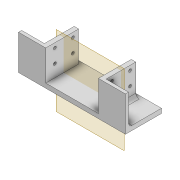
# Autodesk Inventor part: Motor_test_mount
Saved by Autodesk Inventor 2022 (Build 260153000, 153)
## iProperties
Created: 2022-05-04
Part Number: Motor_test_mount
Material: Generic
Document SubType Name: Modeling
Designer: dell
Density: 1 g/cm^3
Appearance: Default
Author: dell
Autodesk Inventor part; units mm, degrees
ref_plane "YZ Plane" through (0, 0, 0) normal (1, 0, 0) x (0, 1, 0)
ref_plane "XZ Plane" through (0, 0, 0) normal (0, 1, 0) x (-1, 0, 0)
ref_plane "XY Plane" through (0, 0, 0) normal (0, 0, 1) x (1, 0, 0)
sketch "Sketch2" plane through (0, 0, 0) normal (1, 0, 0) x (0, 1, 0)
  line L0 (26.4, -3) -> (6, -3)
  line L1 (6, -3) -> (6, -23.4)
  line L2 (6, -23.4) -> (26.4, -23.4)
  line L3 (26.4, -23.4) -> (26.4, -3)
  line L4 (30.4, 0) -> (0, 0)
  line L5 (30.4, -26.4) -> (30.4, 0)
  line L6 (0, 0) -> (0, -26.4)
  line L7 (30.4, -26.4) -> (0, -26.4)
  line L8 (6, -11) -> (0, -11)
  line L9 (0, -11) -> (0, -15.4)
  line L10 (0, -15.4) -> (6, -15.4)
  line L11 (6, -15.4) -> (6, -11)
  point P0 (0, -11)
  dimension "d5" = 20.4
  dimension "d6" = 20.4
  dimension "d8" = 6
  dimension "d22" = 4
  dimension "d23" = 3
  dimension "d24" = 3
  dimension "d27" = 8
  dimension "d28" = 8
  constraints: 24 end point, 4 parallel, 3 horizontal, 2 perpendicular, 2 point on line, 1 coincident, 1 vertical
  measures "d5" distance of L0.start L0.end
  measures "d6" distance of L0.end L1.end
  measures "d8" distance between parallel lines of L1 L6
  measures "d22" distance between parallel lines of L5 L3
  measures "d23" distance between parallel lines of L2 L7
  measures "d24" distance between parallel lines of L4 L0
  measures "d27" distance from line of L0.end L8
  measures "d28" distance from line of L1.end L10
extrude "Extrusion1" add sketch "Sketch2" along normal blind 54.8 contours L0 L1 L8 L6 L4 L5 L7 L10 L2 L3
sketch "Sketch13" plane through (0, 30.4, 0) normal (0, 1, 0) x (1, 0, 0)
  line L0 (0, 0) -> (54.8, 0) projected
  line L1 (0, 26.4) -> (54.8, 26.4) projected
  line L2 (54.8, 0) -> (50.8, 0)
  line L3 (50.8, 0) -> (50.8, 26.4)
  line L4 (50.8, 26.4) -> (54.8, 26.4)
  line L5 (54.8, 26.4) -> (54.8, 0)
  line L6 (4, 0) -> (0, 0)
  line L7 (0, 0) -> (0, 26.4)
  line L8 (0, 26.4) -> (4, 26.4)
  line L9 (4, 26.4) -> (4, 0)
  line L10 (0, 26.4) -> (0, 0) projected
  point P0 (0, 0)
  point P1 (69.8, 0)
  point P2 (69.8, 26.4)
  point P3 (4, 0)
  point P4 (54.8, 26.4)
  point P5 (50.8, 0)
  dimension "d75" = 4
  dimension "d76" = 4
  dimension "d77" = 46.8
  constraints: 17 end point, 4 parallel, 3 point on line, 2 horizontal, 2 perpendicular, 1 collinear
  measures "d75" distance between parallel lines of L5 L3
  measures "d76" distance between parallel lines of L9 L7
  measures "d77" distance between parallel lines of L3 L9
extrude "Extrusion11" add sketch "Sketch13" along normal blind 27 contours L7 L1 L9 L0 | L3 L1 L5 L0
sketch "Sketch14" plane through (54.8, 30.4, 0) normal (1, 0, 0) x (0, 0, -1)
  circle A0 centre (5.2, 11) radius 1.3
  circle A1 centre (5.2, 23) radius 1.3
  line L0 (0, -30.4) -> (0, 27) projected
  circle A2 centre (21.2, 23) radius 1.3
  circle A3 centre (21.2, 11) radius 1.3
  line L1 (26.4, -30.4) -> (26.4, 27) projected
  line L2 (0, 0) -> (26.4, 0) projected
  point P0 (26.4, -4)
  dimension "d80" = 2.6
  dimension "d82" = 2.6
  dimension "d86" = 2.6
  dimension "d87" = 2.6
  dimension "d95" = 16
  dimension "d96" = 16
  dimension "d97" = 5.2
  dimension "d98" = 5.2
  dimension "d99" = 5.2
  dimension "d100" = 5.2
  dimension "d101" = 11
  dimension "d102" = 23
  constraints: 4 centre point
  measures "d80" diameter of A0
  measures "d82" diameter of A1
  measures "d86" diameter of A2
  measures "d87" diameter of A3
  measures "d95" distance of A3.centre A0.centre
  measures "d96" distance of A2.centre A1.centre
  measures "d97" distance from line of L0 A1.centre
  measures "d98" distance from line of L0 A0.centre
  measures "d99" distance from line of L1 A3.centre
  measures "d100" distance from line of L1 A2.centre
  measures "d101" distance from line of L2 A3.centre
  measures "d102" distance from line of A2.centre L2
extrude "Extrusion12" cut sketch "Sketch14" against normal blind 100
ref_plane "Work Plane1" through (0, 0, -13.2) normal (0, 0, 1) x (1, 0, 0)
sketch "Sketch15" plane through (54.8, 0, 0) normal (1, 0, 0) x (0, 0, -1)
  line L0 (3, 26.4) -> (23.4, 26.4) projected
  line L1 (26.4, 30.4) -> (0, 30.4) projected
  line L2 (0, 30.4) -> (26.4, 30.4) projected
  line L3 (-2.8, 30.4) -> (29.2, 30.4)
  line L4 (29.2, 30.4) -> (29.2, 26.4)
  line L5 (29.2, 26.4) -> (-2.8, 26.4)
  line L6 (-2.8, 26.4) -> (-2.8, 30.4)
  line L7 (13.2, -11.48) -> (13.2, 68.88) projected
  line L8 (3, 26.4) -> (23.4, 26.4) projected
  point P0 (0, 0)
  point P1 (13.2, 30.4)
  point P2 (0, 30.4)
  dimension "d103" = 32
  constraints: 8 end point, 2 collinear, 2 parallel, 1 horizontal, 1 midpoint, 1 perpendicular, 1 point on line
  measures "d103" distance between parallel lines of L4 L6
extrude "Extrusion13" add sketch "Sketch15" along normal blind 20 and the other way blind 75
sketch "Sketch16" plane through (-20.2, 30.4, 2.8) normal (0, 1, 0) x (1, 0, 0)
  line L0 (0, 32) -> (0, 0) projected
  line L1 (95, 0) -> (95, 32) projected
  line L2 (0, 0) -> (95, 0)
  line L3 (95, 0) -> (95, 2.8)
  line L4 (95, 2.8) -> (0, 2.8)
  line L5 (0, 2.8) -> (0, 0)
  line L6 (24.2, 29.2) -> (20.2, 29.2) projected
  line L7 (20.2, 29.2) -> (20.2, 2.8) projected
  line L8 (20.2, 2.8) -> (24.2, 2.8) projected
  line L9 (24.2, 2.8) -> (24.2, 29.2) projected
  line L10 (75, 29.2) -> (71, 29.2) projected
  line L11 (71, 29.2) -> (71, 2.8) projected
  line L12 (71, 2.8) -> (75, 2.8) projected
  line L13 (75, 2.8) -> (75, 29.2) projected
  line L14 (0, 0) -> (95, 0) projected
  line L15 (24.2, 2.8) -> (71, 2.8)
  line L16 (71, 2.8) -> (71, 0)
  line L17 (71, 0) -> (24.2, 0)
  line L18 (24.2, 0) -> (24.2, 2.8)
  point P0 (20.2, 2.8)
  point P1 (71, 2.8)
  constraints: 16 end point, 4 parallel, 2 horizontal, 2 perpendicular, 2 point on line
extrude "Extrusion14" add sketch "Sketch16" along normal blind 27 contours L4 L18 L2 L0 | L16 L4 L1 L2
fillet "Fillet5" radius 3 4 edges at (54.8, 30.4, -13.2) (64.8, 30.4, 0) (0, 30.4, -13.2) (-10.1, 30.4, 0)
sketch "Sketch17" plane through (54.8, 0, 0) normal (1, 0, 0) x (0, 0, -1)
  line L0 (-14.3714, 26.4) -> (47.2508, 26.4)
  line L1 (47.2508, 26.4) -> (47.2508, -4.9204)
  line L2 (47.2508, -4.9204) -> (-14.3714, -4.9204)
  line L3 (-14.3714, -4.9204) -> (-14.3714, 26.4)
  line L4 (-2.8, 26.4) -> (29.2, 26.4) projected
  point P0 (0, 0)
  constraints: 8 end point, 2 parallel, 1 collinear, 1 horizontal, 1 perpendicular
extrude "Extrusion15" cut sketch "Sketch17" against normal blind 100
equation "\"d98\" = d97"
body "Solid1"
